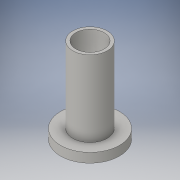
# Autodesk Inventor part: shoulder_washer_plate
Saved by Autodesk Inventor 2016 (Build 200138000, 138)
## iProperties
Created: 2016-02-26
Part Number: shoulder_washer_plate
Material: Generic
Document SubType Name: Modeling
Designer: USKHNGO
Density: 1 g/cm^3
Appearance: Default
Author: USKHNGO
Autodesk Inventor part; units mm, degrees
ref_plane "YZ Plane" through (0, 0, 0) normal (1, 0, 0) x (0, 1, 0)
ref_plane "XZ Plane" through (0, 0, 0) normal (0, 1, 0) x (-1, 0, 0)
ref_plane "XY Plane" through (0, 0, 0) normal (0, 0, 1) x (1, 0, 0)
sketch "Sketch1" plane through (0, 0, 0) normal (0, 1, 0) x (-1, 0, 0)
  circle A0 centre (0, 0) radius 3.683
  circle A1 centre (0, 0) radius 1.778
  dimension "d1" = 7.366
  dimension "d4" = 3.556
  constraints: 2 centre point, 1 coincident
  measures "d1" diameter of A0
  measures "d4" diameter of A1
extrude "Extrusion1" add sketch "Sketch1" along normal blind 10.668
sketch "Sketch2" plane through (0, 10.668, 0) normal (0, 1, 0) x (1, 0, 0)
  circle A0 centre (0, 0) radius 3.683
  circle A1 centre (0, 0) radius 2.159
  dimension "d7" = 4.318
  constraints: 2 centre point, 2 coincident
  measures "d7" diameter of A1
extrude "Extrusion2" cut sketch "Sketch2" against normal blind 9.4996
body "Solid1"
